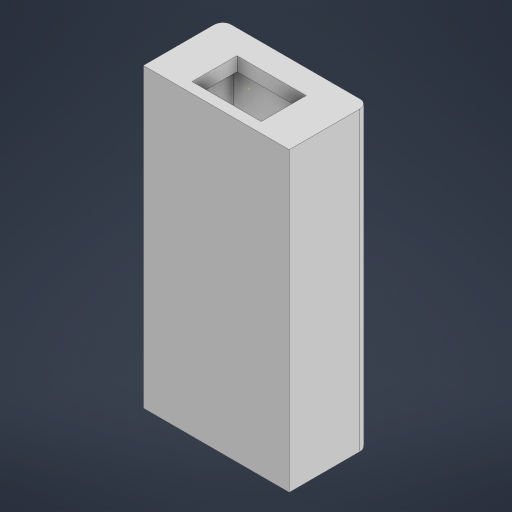
# Autodesk Inventor part: UE306_Sleeve
Saved by Autodesk Inventor 2023 (Build 270158000, 158)
## iProperties
Created: 2023-02-13
Part Number: UE306_Sleeve
Material: Generic
Document SubType Name: Modeling
Designer: uzair
Density: 1 g/cm^3
Appearance: Default
Author: uzair
Autodesk Inventor part; units mm, degrees
ref_plane "YZ Plane" through (0, 0, 0) normal (1, 0, 0) x (0, 1, 0)
ref_plane "XZ Plane" through (0, 0, 0) normal (0, 1, 0) x (-1, 0, 0)
ref_plane "XY Plane" through (0, 0, 0) normal (0, 0, 1) x (1, 0, 0)
sketch "Sketch1" plane through (0, 0, 0) normal (0, 1, 0) x (-1, 0, 0)
  line L0 (36.83, 24.13) -> (-36.83, 24.13)
  line L1 (-36.83, 24.13) -> (-36.83, -24.13)
  line L2 (-36.83, -24.13) -> (36.83, -24.13)
  line L3 (36.83, -24.13) -> (36.83, 24.13)
  line L4 (36.83, 24.13) -> (-36.83, -24.13) construction
  line L5 (-36.83, 24.13) -> (36.83, -24.13) construction
  line L6 (33.02, 21.59) -> (-33.02, 21.59)
  line L7 (-33.02, 21.59) -> (-33.02, -21.59)
  line L8 (-33.02, -21.59) -> (33.02, -21.59)
  line L9 (33.02, -21.59) -> (33.02, 21.59)
  line L10 (33.02, 21.59) -> (-33.02, -21.59) construction
  line L11 (-33.02, 21.59) -> (33.02, -21.59) construction
  point P0 (0, 0)
  dimension "d0" = 73.66
  dimension "d1" = 48.26
  dimension "d2" = 66.04
  dimension "d3" = 43.18
  constraints: 24 end point, 4 midpoint, 4 parallel, 2 horizontal, 2 perpendicular
  measures "d0" distance of L2.end L1.end
  measures "d1" distance of L1.end L0.end
  measures "d2" distance of L8.end L7.end
  measures "d3" distance of L7.end L6.end
extrude "Extrusion1" add sketch "Sketch1" along normal blind 190.5
sketch "Sketch2" plane through (36.83, 0, 24.13) normal (1, 0, 0) x (0, 0, -1)
  line L0 (0, 0) -> (-10.16, 0)
  line L1 (48.26, 0) -> (48.26, 190.5) projected
  line L2 (48.26, 0) -> (58.42, 0)
  line L3 (-10.16, 0) -> (58.42, 0)
  line L4 (58.42, 0) -> (58.42, 190.5)
  line L5 (58.42, 190.5) -> (-10.16, 190.5)
  line L6 (-10.16, 190.5) -> (-10.16, 0)
  line L7 (-10.16, 190.5) -> (58.42, 190.5)
  line L8 (58.42, 190.5) -> (58.42, 200.66)
  line L9 (58.42, 200.66) -> (-10.16, 200.66)
  line L10 (-10.16, 200.66) -> (-10.16, 190.5)
  line L11 (0, 190.5) -> (48.26, 190.5) projected
  line L12 (-10.16, 0) -> (0, 0)
  line L13 (0, 0) -> (0, 190.5)
  line L14 (0, 190.5) -> (-10.16, 190.5)
  line L15 (-10.16, 190.5) -> (-10.16, 0)
  line L16 (0, 190.5) -> (58.42, 190.5)
  line L17 (58.42, 190.5) -> (58.42, 200.66)
  line L18 (58.42, 200.66) -> (0, 200.66)
  line L19 (0, 200.66) -> (0, 190.5)
  point P0 (24.13, 0)
  dimension "d6" = 10.16
  dimension "d7" = 10.16
  dimension "d8" = 10.16
  constraints: 36 end point, 8 parallel, 6 horizontal, 4 perpendicular
  measures "d6" distance of L0.start L0.end
  measures "d7" distance of L1.start L2.end
  measures "d8" distance of L8.end L7.end
extrude "Extrusion2" add sketch "Sketch2" against normal blind 90.5129 contours L1 L5 L4 L2 | L19 L9 L8 L5
extrude "Extrusion3" add sketch "Sketch2" along normal blind 16.8529 contours L1 L5 L4 L2 | L19 L9 L8 L5
sketch "Sketch3" plane through (-33.02, 190.5, 21.59) normal (0, -1, 0) x (1, 0, 0)
  line L0 (66.04, 0) -> (0, 0) projected
  line L1 (0, -43.18) -> (66.04, -43.18) projected
  line L2 (66.04, 0) -> (0, 0)
  line L3 (0, 0) -> (0, -43.18)
  line L4 (0, -43.18) -> (66.04, -43.18)
  line L5 (66.04, -43.18) -> (66.04, 0)
  line L6 (58.42, -5.08) -> (7.62, -5.08)
  line L7 (7.62, -5.08) -> (7.62, -38.1)
  line L8 (7.62, -38.1) -> (58.42, -38.1)
  line L9 (58.42, -38.1) -> (58.42, -5.08)
  line L10 (58.42, -5.08) -> (7.62, -38.1) construction
  line L11 (7.62, -5.08) -> (58.42, -38.1) construction
  point P0 (33.02, -21.59)
  dimension "d13" = 50.8
  dimension "d14" = 33.02
  constraints: 20 end point, 4 parallel, 2 horizontal, 2 midpoint, 2 perpendicular
  measures "d13" distance of L8.end L7.end
  measures "d14" distance of L7.end L6.end
extrude "Extrusion4" cut sketch "Sketch3" against normal blind 10.16 contours L9 L8 L7 L6
sketch "Sketch4" plane through (36.83, 0, -24.13) normal (0, 0, 1) x (1, 0, 0)
  line L0 (16.8529, 190.5) -> (16.8529, 0) projected
  line L1 (0, 0) -> (0, 190.5) projected
  line L2 (16.8529, 0) -> (0, 0)
  line L3 (0, 0) -> (0, 190.5)
  line L4 (0, 190.5) -> (16.8529, 190.5)
  line L5 (16.8529, 190.5) -> (16.8529, 0)
  line L6 (-73.66, 190.5) -> (-90.5129, 190.5) projected
  line L7 (-90.5129, 0) -> (-90.5129, 190.5) projected
  line L8 (-73.66, 190.5) -> (-90.5129, 190.5)
  line L9 (-90.5129, 190.5) -> (-90.5129, 0)
  line L10 (-90.5129, 0) -> (-73.66, 0)
  line L11 (-73.66, 0) -> (-73.66, 190.5)
  point P0 (-36.83, 0)
  constraints: 16 end point, 4 parallel, 2 horizontal, 2 perpendicular
extrude "Extrusion5" add sketch "Sketch4" along normal blind 48.26
sketch "Sketch5" plane through (-53.6829, 200.66, 24.13) normal (0, 1, 0) x (1, 0, 0)
  point P0 (53.6829, 24.13)
sketch "Sketch6" plane through (0, 0, 0) normal (0, -1, 0) x (1, 0, 0)
  line L0 (-53.6829, 24.13) -> (53.6829, 24.13) projected
  line L1 (-53.6829, -34.29) -> (53.6829, -34.29) projected
  line L2 (-53.6829, 24.13) -> (53.6829, 24.13)
  line L3 (53.6829, 24.13) -> (53.6829, -34.29)
  line L4 (53.6829, -34.29) -> (-53.6829, -34.29)
  line L5 (-53.6829, -34.29) -> (-53.6829, 24.13)
  line L6 (33.02, 21.59) -> (-33.02, 21.59) projected
  line L7 (33.02, -21.59) -> (33.02, 21.59) projected
  line L8 (-33.02, 21.59) -> (33.02, 21.59)
  line L9 (33.02, 21.59) -> (33.02, -21.59)
  line L10 (33.02, -21.59) -> (-33.02, -21.59)
  line L11 (-33.02, -21.59) -> (-33.02, 21.59)
  point P0 (0, 0)
  constraints: 16 end point, 4 parallel, 2 horizontal, 2 perpendicular
extrude "Extrusion6" add sketch "Sketch6" along normal blind 17.7038
fillet "Fillet1" radius 6.3754 2 edges at (53.6829, 91.4781, -34.29) (-53.6829, 91.4781, -34.29)
body "Solid1"
